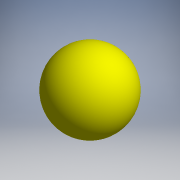
# Autodesk Inventor part: SKF_6003-2Z_PART3
Saved by Autodesk Inventor 2017.3 (Build 213256000, 256)
## iProperties
Part Number: SKF_6003-2Z_PART3
Material: Generic
Catalog Web Link: www.cadenas.de
Description: -Deep groove ball bearings
Vendor: SKF
Document SubType Name: Modeling
Designer: partserver
Manufacturer: SKF
Mass: 41 g
Surface Area: 0.712408 cm^2
Volume: 0.0565414 cm^3
Density: 1 g/cm^3
Appearance: PSOLRGB-192-192-192
Category: PARTsolutions
Company: SKF
Title: SKF_6003-2Z_PART3
Author: Cadenas PARTsolutions
Comments: Deep groove ball bearings
PSOL_IDENT_0: {$CADENAS_DATA\23d-libs\skf\bearings_units_and_housings\ball_bearings\deep_groove_ball_bearings\bb1_
PSOL_IDENT_1: 001_101.prj},200 {VTYP=3D},{NB=SKF_6003-2Z_PART3},{LINA=SKF_6003-2Z_PART3},{NN=BB1_001_101_PART3},{N
PSOL_IDENT_2: OPRJ=TRUE},{DATE=08.10.2021 05:14:16},{GEOMDATE=07.09.2021 05:54:21},{VERSION=},{LINEID=4560},{WBVAR=
PSOL_IDENT_3: },{WBNUMERIC=}  {NB=SKF_6003-2Z_PART3},{LINA=SKF_6003-2Z_PART3},{KT=DUMMY},{DESIGNATION=6003-2Z},{R1
PSOL_IDENT_4: 2=0.30},{DD=17.000},{D=35.000},{B=10.000},{C=},{CX=},{CXX=},{CA=0.000},{XXVARIANT=},{XXDESIGN=Single
PSOL_IDENT_5: row},{XXSEALING=Shield on both sides},{DESIGN=dgbbw2z},{DESIGNIR=dgbbw2z},{VARIANT=},{DD1=23.00},{D
PSOL_IDENT_6: D2=},{DD2X=},{DD2A=0.00},{D1=29.20},{D1X=MIN},{D2=31.2},{D2A=31.20},{D3=},{D3X=},{D3A=0.000},{D4=},{
PSOL_IDENT_7: HH=MIN},{BB=MIN},{BBX=},{BBA=0.000},{FF=},{R0MAX=MIN},{R0=MIN},{PITCH=26.00},{DW=4.762},{DDAMIN=19.0
PSOL_IDENT_8: 00},{DDAMAX=22.900},{DDBMIN=MIN},{DDBMAX=MIN},{DBMIN=MIN},{DAMAX=33.000},{BBAMIN=MIN},{CAMAX=MIN},{R
PSOL_IDENT_9: AMAX=0.300},{LOAD1=6.370},{LOAD2=3.250},{LOAD3=0.137},{SPEED1=45000},{SPEED2=22000},{KR=0.025},{F0=1
PSOL_IDENT_10: 4.000},{Z=10},{II=1},{MASS=0.041},{BEARING=6003-2Z},{RING=},{HELP=2.900},{HELP2=1.900},{DD1ALG=11.50
PSOL_IDENT_11: 0},{YALG=11.500},{PITCH1=26.000},{DW1=4.762},{YALG1=14.600},{HALG1=2.900},{SH=11.500},{CU=1.048},{HA
PSOL_IDENT_12: LG=3},{B1=0},{SHIELDHELP=2},{D4A=0.000},{FFA=0.000},{RS1=}
NB: SKF_6003-2Z_PART3
NT: Deep groove ball bearings
NBSYN: SKF_$DESIGNATION._PART3
LINA: SKF_6003-2Z_PART3
CATALOG: SKF
DESIGNATION: 6003-2Z
R12: 0.3
DD: 17
D: 35
B: 10
D2: 31.2
LOAD1: 6.37
LOAD2: 3.25
LOAD3: 0.137
SPEED1: 45000
SPEED2: 22000
BEARING: 6003-2Z
SUPPLIER: SKF
ARTICLENO: SKF_6003-2Z_PART3
BOMINFO: SKF_6003-2Z_PART3
CREATOR: CADENAS GmbH
Autodesk Inventor part; units mm, degrees
ref_plane "YZ Plane" through (0, 0, 0) normal (1, 0, 0) x (0, 1, 0)
ref_plane "XZ Plane" through (0, 0, 0) normal (0, 1, 0) x (-1, 0, 0)
ref_plane "XY Plane" through (0, 0, 0) normal (0, 0, 1) x (1, 0, 0)
sketch "Sketch_6" plane through (0, 0, 0) normal (0, 0, 1) x (1, 0, 0)
  line L0 (7.381, 13) -> (2.619, 13)
  arc A0 (7.381, 13) -> (2.619, 13) centre (5, 13) ccw
  line L1 (7.381, 13) -> (2.619, 13)
  dimension "d0" = 360
  constraints: 4 end point, 2 point on circle, 1 centre point
revolve "Revolution1" add sketch "Sketch_6" angle 360 about axis through (7.381, 13, 0) along (1, 0, 0)
body "Solid1"
